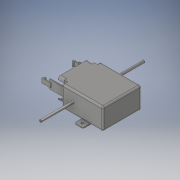
# Autodesk Inventor part: Part4
Saved by Autodesk Inventor 2019 (Build 230136000, 136)
## iProperties
Created: 2019-08-08
Part Number: Part4
Material: Iron, Malleable
Document SubType Name: Modeling
Designer: daozhou.cen
Density: 7.15 g/cm^3
Appearance: Semi-Polished
Author: daozhou.cen
Autodesk Inventor part; units mm, degrees
ref_plane "YZ Plane" through (0, 0, 0) normal (1, 0, 0) x (0, 1, 0)
sketch "Sketch1" plane through (0, 0, 0) normal (0, 0, 1) x (1, 0, 0)
  circle A0 centre (0, 0) radius 1.45
  dimension "d0" = 2.9
  constraints: 1 centre point, 1 coincident
  measures "d0" diameter of A0
extrude "Extrusion1" add sketch "Sketch1" along normal blind 120
sketch "Sketch2" plane through (0, 0, 0) normal (1, 0, 0) x (0, 1, 0)
  line L0 (1.45, 120) -> (-1.45, 120) projected
  line L1 (-1.45, 0) -> (1.45, 0) projected
  line L2 (1.45, 0) -> (1.45, 120) projected
  line L3 (-1.45, 0) -> (-1.45, 120) projected
  line L4 (1.45, 0) -> (-1.45, 120) construction
  line L5 (1.45, 120) -> (-1.45, 0) construction
  line L6 (12.5, 37.5) -> (-12.5, 37.5)
  line L7 (-12.5, 37.5) -> (-12.5, 82.5)
  line L8 (-12.5, 82.5) -> (12.5, 82.5)
  line L9 (12.5, 82.5) -> (12.5, 37.5)
  line L10 (12.5, 37.5) -> (-12.5, 82.5) construction
  line L11 (-12.5, 37.5) -> (12.5, 82.5) construction
  line L12 (12.5, 42.5) -> (-12.5, 42.5)
  line L13 (-12.5, 42.5) -> (-12.5, 77.5)
  line L14 (-12.5, 77.5) -> (12.5, 77.5)
  line L15 (12.5, 77.5) -> (12.5, 42.5)
  line L16 (12.5, 42.5) -> (-12.5, 77.5) construction
  line L17 (-12.5, 42.5) -> (12.5, 77.5) construction
  point P0 (0, 60)
  dimension "d3" = 25
  dimension "d4" = 45
  dimension "d7" = 25
  dimension "d8" = 35
  constraints: 28 end point, 5 midpoint, 4 parallel, 2 horizontal, 2 perpendicular
  measures "d3" distance of L7.end L8.end
  measures "d4" distance of L6.end L7.end
  measures "d7" distance of L13.end L14.end
  measures "d8" distance of L12.end L13.end
extrude "Extrusion2" add sketch "Sketch2" along normal blind 35 separate body contours L8 L9 L14 L2 | L2 L14 L3 L8 | L3 L14 L7 L8 | L14 L9 L12 L2 | L2 L12 L3 L14 | L3 L12 L7 L14 | L12 L9 L6 L2 | L2 L6 L3 L12 | L3 L6 L7 L12
extrude "Extrusion3" add sketch "Sketch2" against normal blind 15 contours L14 L9 L12 L2 | L2 L12 L3 L14 | L3 L12 L7 L14 bodies 2
sketch "Sketch3" plane through (-15, 0, 0) normal (-1, 0, 0) x (0, 0, 1)
  line L0 (42.5, 12.5) -> (42.5, -12.5) construction
  line L1 (37.5, -12.5) -> (82.5, -12.5) construction
  line L2 (42.5, 12.5) -> (77.5, 12.5) construction
  line L3 (77.5, 12.5) -> (77.5, -12.5) construction
  line L4 (77.5, -12.5) -> (42.5, -12.5) construction
  line L5 (42.5, -12.5) -> (42.5, 12.5) construction
  line L6 (77.5, 12.5) -> (77.5, -12.5) construction
  line L7 (42.5, 12.5) -> (77.5, 12.5) construction
  line L8 (77.5, 12.5) -> (77.5, 9.5) construction
  line L9 (77.5, 9.5) -> (42.5, 9.5) construction
  line L10 (42.5, 9.5) -> (42.5, 12.5) construction
  line L11 (77.5, 12.5) -> (77.5, -12.5) construction
  line L12 (42.5, -12.5) -> (77.5, -12.5) construction
  line L13 (77.5, -12.5) -> (77.5, -9.5) construction
  line L14 (77.5, -9.5) -> (42.5, -9.5) construction
  line L15 (42.5, -9.5) -> (42.5, -12.5) construction
  arc A0 (45.5, 12.5) -> (42.5, 9.5) centre (45.5, 9.5) ccw
  arc A1 (77.5, 9.5) -> (74.5, 12.5) centre (74.5, 9.5) ccw
  line L16 (45.5, 12.5) -> (74.5, 12.5)
  line L17 (37.5, 12.5) -> (82.5, 12.5) projected
  arc A2 (42.5, -9.5) -> (45.5, -12.5) centre (45.5, -9.5) ccw
  arc A3 (74.5, -12.5) -> (77.5, -9.5) centre (74.5, -9.5) ccw
  line L18 (45.5, -12.5) -> (74.5, -12.5)
  line L19 (42.5, 9.5) -> (43.5, 9.5)
  line L20 (77.5, 9.5) -> (76.5, 9.5)
  arc A4 (45.5, 11.5) -> (43.5, 9.5) centre (45.5, 9.5) ccw
  arc A5 (76.5, 9.5) -> (74.5, 11.5) centre (74.5, 9.5) ccw
  line L21 (74.5, 11.5) -> (45.5, 11.5)
  line L22 (42.5, -9.5) -> (43.5, -9.5)
  line L23 (77.5, -9.5) -> (76.5, -9.5)
  arc A6 (43.5, -9.5) -> (45.5, -11.5) centre (45.5, -9.5) ccw
  arc A7 (74.5, -11.5) -> (76.5, -9.5) centre (74.5, -9.5) ccw
  line L24 (74.5, -11.5) -> (45.5, -11.5)
  line L25 (42.5, 5) -> (43.5, 5)
  line L26 (43.5, 5) -> (43.5, -5)
  line L27 (43.5, -5) -> (42.5, -5)
  line L28 (42.5, -5) -> (42.5, 5)
  line L29 (42.5, 5) -> (43.5, -5) construction
  line L30 (43.5, 5) -> (42.5, -5) construction
  line L31 (77.5, -12.5) -> (77.5, 12.5) projected
  line L32 (76.5, 5) -> (77.5, 5)
  line L33 (77.5, 5) -> (77.5, -5)
  line L34 (77.5, -5) -> (76.5, -5)
  line L35 (76.5, -5) -> (76.5, 5)
  line L36 (76.5, 5) -> (77.5, -5) construction
  line L37 (77.5, 5) -> (76.5, -5) construction
  line L38 (42.5, 0) -> (77.5, 0) construction
  line L39 (42.5, 9.5) -> (43.5, 9.5) construction
  line L40 (43.5, 9.5) -> (43.5, -9.5) construction
  line L41 (43.5, -9.5) -> (42.5, -9.5) construction
  line L42 (42.5, -9.5) -> (42.5, 9.5) construction
  point P0 (0, 0)
  point P1 (77.5, 1.45)
  point P2 (77.5, -1.45)
  point P3 (43, 0)
  point P4 (77, 0)
  point P5 (43, 0)
  dimension "d11" = 3
  dimension "d12" = 3
  dimension "d13" = 1
  dimension "d14" = 1
  dimension "d15" = 1
  dimension "d16" = 1
  dimension "d17" = 1
  dimension "d18" = 1
  dimension "d21" = 10
  dimension "d22" = 10
  dimension "d23" = 35
  dimension "d24" = 17.5
  dimension "d25" = 32
  constraints: 74 end point, 17 point on circle, 15 parallel, 15 point on line, 11 tangent, 8 centre point, 7 horizontal, 7 midpoint, 6 perpendicular, 3 collinear, 2 concentric, 2 other
  measures "d11" distance of L7.end L8.end
  measures "d12" distance of L13.end L12.end
  measures "d13" distance of L9.end L19.end
  measures "d14" distance of L8.end L20.end
  measures "d15" distance of L14.end L22.end
  measures "d16" distance of L13.end L23.end
  measures "d17" distance from line of L4 L24.end
  measures "d18" distance between parallel lines of L21 L16
  measures "d21" distance of L25.end L26.end
  measures "d22" distance of L32.end L33.end
  measures "d23" distance between parallel lines of L6 L28
  measures "d24" distance between parallel lines of L17 L34
  measures "d25" distance from line of A4.start L11
extrude "Extrusion4" add sketch "Sketch3" along normal blind 7 contours L16 A1 L20 A5 L21 A4 L19 A0 | A3 L18 A2 L22 A6 L24 A7 L23 bodies 2
extrude "Extrusion5" add sketch "Sketch3" along normal blind 17 contours L31 L34 L35 L32 | L25 L26 L27 L28 bodies 2
sketch "Sketch5" plane through (-15, 12.5, 77.5) normal (0, 0, 1) x (1, 0, 0)
  line L0 (-25, -10) -> (-15, -10) construction
  line L1 (-15, -10) -> (-15, -15) construction
  line L2 (-15, -15) -> (-25, -15) construction
  line L3 (-25, -15) -> (-25, -10) construction
  line L4 (-25, -10) -> (-15, -15) construction
  line L5 (-15, -10) -> (-25, -15) construction
  line L6 (0, -17.5) -> (0, -7.5) construction
  line L7 (-25, -10) -> (-15, -10)
  line L8 (-15, -10) -> (-15, -15)
  line L9 (-15, -15) -> (-25, -15)
  line L10 (-25, -15) -> (-25, -10)
  point P0 (15, -12.5)
  point P1 (-20, -12.5)
  dimension "d28" = 10
  dimension "d29" = 5
  dimension "d32" = 15
  constraints: 20 end point, 4 parallel, 2 horizontal, 2 midpoint, 2 perpendicular
  measures "d28" distance of L1.end L2.end
  measures "d29" distance of L0.end L1.end
  measures "d32" distance between parallel lines of L6 L1
extrude "Extrusion6" add sketch "Sketch5" along normal blind 1 bodies 2
sketch "Sketch6" plane through (0, -12.5, 42.5) normal (0, 0, -1) x (-1, 0, 0)
  line L0 (40, 15) -> (30, 15) projected
  line L1 (40, 10) -> (40, 15) projected
  line L2 (32, 10) -> (40, 10) projected
  line L3 (30, 15) -> (30, 10) projected
  line L4 (30, 10) -> (32, 10) projected
  point P0 (0, 12.5)
extrude "Extrusion7" add sketch "Sketch6" along normal blind 1 bodies 2
extrude "Extrusion8" add sketch "Sketch2" against normal blind 13 contours L8 L9 L14 L2 | L2 L14 L3 L8 | L3 L14 L7 L8 | L14 L9 L12 L2 | L2 L12 L3 L14 | L3 L12 L7 L14 | L12 L9 L6 L2 | L2 L6 L3 L12 | L3 L6 L7 L12 bodies 2
extrude "Extrusion9" cut sketch "Sketch2" against normal blind 13 contours L14 L9 L12 L2 | L2 L12 L3 L14 | L3 L12 L7 L14 bodies 1
sketch "Sketch11" plane through (0, -1.45, 42.5) normal (0, 0, 1) x (1, 0, 0)
  arc A0 (0, 2.9) -> (0, 0) centre (0, 1.45) ccw projected
  line L0 (0, 2.9) -> (0, 0) projected
extrude "Extrusion12" add sketch "Sketch11" along normal up to surface (35 mm away) bodies 1
sketch "Sketch9" plane through (0, -12.5, 42.5) normal (0, 0, 1) x (1, 0, 0)
  line L0 (-40, 10) -> (-40, 15) projected
  line L1 (-40, 15) -> (-30, 15) projected
  line L2 (-40, 10) -> (-38, 10)
  line L3 (-38, 10) -> (-38, 15)
  line L4 (-38, 15) -> (-40, 15)
  line L5 (-40, 15) -> (-40, 10)
  point P0 (0, 12.5)
  dimension "d43" = 2
  constraints: 8 end point, 2 parallel, 1 horizontal, 1 perpendicular, 1 point on line
  measures "d43" distance of L4.end L3.end
extrude "Extrusion10" add sketch "Sketch9" along normal blind 2 bodies 2
sketch "Sketch10" plane through (-15, 12.5, 77.5) normal (0, 0, -1) x (-1, 0, 0)
  line L0 (25, -15) -> (23, -15) projected
  line L1 (23, -15) -> (23, -10) projected
  line L2 (23, -10) -> (25, -10) projected
  line L3 (25, -10) -> (25, -15) projected
  point P0 (-15, -12.5)
extrude "Extrusion11" add sketch "Sketch10" along normal blind 2 bodies 2
fillet "Fillet1" radius 2 2 edges at (-40, 0, 75.5) (-40, 0, 44.5)
fillet "Fillet5" radius 2 14 edges at (11, 12.5, 82.5) (-13, 0, 82.5) (11, -12.5, 82.5) (35, 0, 82.5) (35, 12.5, 60) (35, -12.5, 60) (35, 0, 37.5) (11, 12.5, 37.5) (11, -12.5, 37.5) (-13, 0, 37.5) (-13, 12.5, 40) (-13, -12.5, 40) (-13, -12.5, 80) (-13, 12.5, 80)
ref_plane "Work Plane1" through (-13, -6.25, 39.5) normal (0, 0, -1) x (0, 1, 0)
sketch "Sketch14" plane through (-13, -6.25, 39.5) normal (0, 0, -1) x (0, 1, 0)
  line L0 (-6.25, 2) -> (-6.25, 46) projected
  line L1 (-6.25, 33) -> (-5.25, 33)
  line L2 (-5.25, 33) -> (-5.25, 23)
  line L3 (-5.25, 23) -> (-6.25, 23)
  line L4 (-6.25, 23) -> (-6.25, 33)
  line L5 (-4.25, 48) -> (16.75, 48) projected
  point P0 (6.25, 13)
  dimension "d63" = 1
  dimension "d64" = 10
  dimension "d68" = 15
  constraints: 8 end point, 2 parallel, 1 horizontal, 1 perpendicular, 1 point on line
  measures "d63" distance of L2.end L3.end
  measures "d64" distance of L1.end L2.end
  measures "d68" distance between parallel lines of L1 L5
extrude "Extrusion14" add sketch "Sketch14" along normal blind 10 bodies 2
fillet "Fillet7" radius 2 2 edges at (20, -12, 29.5) (10, -12, 29.5)
ref_plane "Work Plane2" through (35, 6.25, 80.5) normal (0, 0, 1) x (0, 1, 0)
sketch "Sketch15" plane through (35, 6.25, 80.5) normal (0, 0, 1) x (0, 1, 0)
  line L0 (-17.75, 15) -> (-18.75, 15) projected
  line L1 (-18.75, 17) -> (-18.75, 23) projected
  line L2 (-18.75, 15) -> (-18.75, 17) projected
  line L3 (-17.75, 17) -> (-17.75, 15) projected
  line L4 (-17.75, 23) -> (-17.75, 17) projected
  line L5 (-17.75, 25) -> (-17.75, 23) projected
  line L6 (-18.75, 25) -> (-17.75, 25) projected
  line L7 (-18.75, 23) -> (-18.75, 25) projected
  line L8 (-18.75, 46) -> (-18.75, 2) projected
  point P0 (-6.25, 35)
extrude "Extrusion15" add sketch "Sketch15" along normal blind 10 bodies 2
fillet "Fillet8" radius 2 2 edges at (20, -12, 90.5) (10, -12, 90.5)
sketch "Sketch16" plane through (10, -11.5, 37.7679) normal (0, 1, 0) x (1, 0, 0)
  line L0 (0, 0) -> (0, 6.2679) projected
  line L1 (10, 0) -> (10, 6.2679) projected
  line L2 (23, 0.2679) -> (-21, 0.2679) projected
  line L3 (2, 8.2679) -> (8, 8.2679) projected
  point P0 (-10, 37.7679)
  point P1 (5, 4.2679)
  dimension "d72" = 10
  dimension "d73" = 5
  dimension "d74" = 8
  dimension "d75" = 4
  measures "d72" distance between parallel lines of L0 L1
  measures "d73" distance from line of point (5, 4.268) L1
  measures "d74" distance between parallel lines of L2 L3
  measures "d75" distance from line of point (5, 4.268) L3
hole "Hole1" at (15, -11.5, 33.5) direction (0, -1, 0) diameter 2.5 end through all bodies 2
sketch "Sketch17" plane through (10, -11.5, 82.2321) normal (0, 1, 0) x (1, 0, 0)
  line L0 (10, 0) -> (10, -6.2679) projected
  line L1 (0, 0) -> (0, -6.2679) projected
  line L2 (-21, -0.2679) -> (23, -0.2679) projected
  line L3 (8, -8.2679) -> (2, -8.2679) projected
  point P0 (-10, 82.2321)
  point P1 (5, -4.2679)
  dimension "d83" = 10
  dimension "d84" = 5
  dimension "d85" = 8
  dimension "d86" = 4
  measures "d83" distance between parallel lines of L0 L1
  measures "d84" distance from line of point (5, -4.268) L1
  measures "d85" distance between parallel lines of L2 L3
  measures "d86" distance from line of L3 point (5, -4.268)
hole "Hole2" at (15, -11.5, 86.5) direction (0, -1, 0) diameter 2.5 end through all bodies 2
equation "\"d73\" = 0.5 * d72"
equation "\"d75\" = 0.5 * d74"
equation "\"d84\" = 0.5 * d83"
equation "\"d86\" = 0.5 * d85"
body "Solid1"
body "Solid3"
